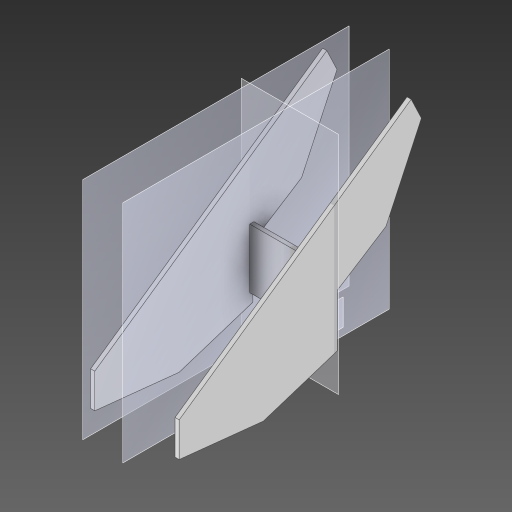
# Autodesk Inventor part: ShoulderBoundingBox
Saved by Autodesk Inventor 2023 (Build 270158000, 158)
## iProperties
Created: 2023-03-18
Part Number: ShoulderBoundingBox
Material: Generic
Document SubType Name: Modeling
Designer: Val
Density: 1 g/cm^3
Appearance: Default
Author: Val
Autodesk Inventor part; units mm, degrees
ref_plane "XZ Plane" through (0, 0, 0) normal (0, 1, 0) x (-1, 0, 0)
ref_plane "Work Plane1" through (30.48, 0, 0) normal (1, 0, 0) x (0, 1, 0)
sketch "Sketch1" plane through (30.48, 0, 0) normal (1, 0, 0) x (0, 1, 0)
  line L0 (-20.1241, -2.3129) -> (-38.2674, 53.7867)
  line L1 (-38.2674, 53.7867) -> (-31.5623, 117.8336)
  line L2 (-31.5623, 117.8336) -> (-5.4691, 117.8336)
  line L3 (-5.4691, 117.8336) -> (117.3937, -58.5065)
  line L4 (117.3937, -58.5065) -> (101.0815, -66.2557)
  line L5 (19.6952, -2.3129) -> (-20.1241, -2.3129)
  line L6 (101.0815, -66.2557) -> (43.3079, -39.3441)
  line L7 (43.3079, -39.3441) -> (19.6952, -2.3129)
  line L8 (-37.8354, 57.9131) -> (-33.5614, 98.738)
  point P0 (0, 0)
  point P1 (-12.6907, 108.8336)
  point P2 (0, 0)
  dimension "d1" = 9
  dimension "d2" = 39.8192
  dimension "d3" = 107.922
  dimension "d5" = 56.0996
  dimension "d6" = 84.023
  dimension "d7" = 64.0469
  dimension "d8" = 26.0932
  dimension "d9" = 55.134
  dimension "d10" = 176.3401
  dimension "d11" = 37.0312
  dimension "d12" = 26.9116
  dimension "d13" = 18.8716
  dimension "d14" = 111.1466
  constraints: 18 end point, 2 collinear, 2 horizontal, 1 other
  measures "d1" distance from line of L2 point (-12.691, 108.834)
  measures "d2" distance of L5.start L0.start
  measures "d3" angle of L0 L5
  measures "d5" vertical distance of L0.start L0.end
  measures "d6" angle of L8 L5
  measures "d7" vertical distance of L0.end L2.start
  measures "d8" distance of L2.start L3.start
  measures "d9" angle of L3 L5
  measures "d10" vertical distance of L3.start L4.start
  measures "d11" vertical distance of L7.start L5.start
  measures "d12" vertical distance of L6.start L7.start
  measures "d13" horizontal distance of L2.start point (-12.691, 108.834)
  measures "d14" distance from line of L5 point (-12.691, 108.834)
extrude "Extrusion1" add sketch "Sketch1" along normal blind 3.175
ref_plane "Work Plane2" through (-30.48, 0, 0) normal (1, 0, 0) x (0, 1, 0)
sketch "Sketch2" plane through (-30.48, 0, 0) normal (1, 0, 0) x (0, 1, 0)
  line L0 (-20.1241, -2.3129) -> (19.6952, -2.3129) projected
  line L1 (19.6952, -2.3129) -> (43.3079, -39.3441) projected
  line L2 (43.3079, -39.3441) -> (101.0815, -66.2557) projected
  line L3 (101.0815, -66.2557) -> (117.3937, -58.5065) projected
  line L4 (117.3937, -58.5065) -> (-5.4691, 117.8336) projected
  line L5 (-5.4691, 117.8336) -> (-31.5623, 117.8336) projected
  line L6 (-31.5623, 117.8336) -> (-38.2674, 53.7867) projected
  line L7 (-38.2674, 53.7867) -> (-20.1241, -2.3129) projected
  point P0 (0, 0)
extrude "Extrusion2" add sketch "Sketch2" against normal blind 3.175
sketch "Sketch3" plane through (0, 0, 0) normal (0, 0, 1) x (1, 0, 0)
  line L0 (-30.48, -12.7) -> (30.48, -12.7)
  line L1 (30.48, -12.7) -> (30.48, 32.385)
  line L2 (30.48, 32.385) -> (-30.48, 32.385)
  line L3 (-30.48, 32.385) -> (-30.48, -12.7)
  line L4 (-30.48, 117.3937) -> (-30.48, -5.4691) projected
  line L5 (30.48, 117.3937) -> (30.48, -5.4691) projected
  point P0 (0, 0)
  dimension "d20" = 12.7
  dimension "d21" = 32.385
  constraints: 8 end point, 2 collinear, 2 parallel, 1 horizontal, 1 perpendicular
  measures "d20" distance from line of L0 point (0, 0)
  measures "d21" distance from line of L2 point (0, 0)
extrude "Extrusion3" add sketch "Sketch3" against normal blind 3.175
body "Solid1"
